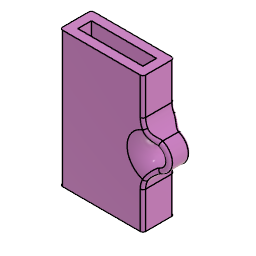
Ear Silent Slider v3 (Autodesk Fusion 360 design; units mm, degrees)
Autodesk Fusion 360 part; units mm, degrees
sketch "Sketch1" plane through (0, 0, 0) normal (0, 0, 1) x (1, 0, 0)
  line L0 (0, 0) -> (-7.2, 0)
  line L1 (-7.2, 0) -> (-7.2, 1.5)
  line L2 (-7.2, 1.5) -> (0, 1.5)
  line L3 (0, 1.5) -> (0, 0)
  dimension "d1" = 7.2
  dimension "d2" = 1.5
  constraint horizontal L0
  constraint vertical L1
  constraint horizontal L2
  constraint vertical L3
  constraint coincident L0.start L3.end
  measures "d1" distance of L0.start L0.end
  measures "d2" distance of L0.end L1.end
extrude "Extrude1" add sketch "Sketch1" along normal mid plane 15 thin wall 1 on the left open curves L2 L3 L0 L1
sketch "Sketch2" plane through (0, 0, 0) normal (0, 1, 0) x (1, 0, 0)
  line L0 (1, -7.5) -> (1, 7.5)
  circle A0 centre (1.75, 0) radius 0.75
  circle A1 centre (1.75, 0) radius 1.65
  line L1 (1.75, -1.65) -> (1, -1.65)
  line L2 (1.75, 1.65) -> (1, 1.65)
  dimension "d6" = 0.9
  dimension "d7" = 1.5
  constraint horizontal origin A0.centre
  constraint coincident A1 L1.start
  constraint coincident L0 L1.end
  constraint perpendicular L0 L1
  constraint coincident A1 L2.start
  constraint coincident L0 L2.end
  constraint perpendicular L0 L2
  constraint tangent A1 L2
  constraint tangent A1 L1
  constraint tangent L0 A0
  measures "d7" diameter of A0
extrude "Extrude2" add sketch "Sketch2" along normal up to surface (-1 mm away) and the other way up to surface (-2.5 mm away)
fillet "Fillet1" radius 2 2 edges at (1, 0.75, 1.65) (1, 0.75, -1.65)
fillet "Fillet3" radius 1.75 2 edges at (1.0508, -1, -0.2712) (1.0508, 2.5, 0.2712)
fillet "Fillet2" radius 0.3 16 edges at (1, 2.5, 5.4646) (1.065, 2.5, 2.9235) (1.6951, 2.3991, 1.9136) (3.4, 2.2797, 0) (1.7708, 2.3754, -1.8516) (1.065, 2.5, -2.9235) (1, 2.5, -5.4646) (1, -1, 5.4646) (1.065, -1, 2.9235) (1.7771, -0.8735, 1.8467) (3.4, -0.7797, 0) (1.6595, -0.9104, -1.945) (1.065, -1, -2.9235) (1, -1, -5.4646) (-8.2, 2.5, 0) (-8.2, -1, 0)
equation "d3 = 1.00 mm"
equation "d17 = ( d2 + 2 * d3 ) / 2"
